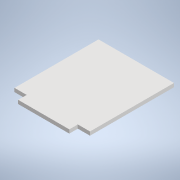
# Autodesk Inventor part: divider 2
Saved by Autodesk Inventor 2022 (Build 260153000, 153)
## iProperties
Created: 2022-05-12
Part Number: divider 2
Material: Generic
Document SubType Name: Modeling
Designer: Jeanette Guo
Density: 1 g/cm^3
Appearance: Default
Author: Jeanette Guo
Autodesk Inventor part; units mm, degrees
ref_plane "YZ Plane" through (0, 0, 0) normal (1, 0, 0) x (0, 1, 0)
ref_plane "XZ Plane" through (0, 0, 0) normal (0, 1, 0) x (-1, 0, 0)
ref_plane "XY Plane" through (0, 0, 0) normal (0, 0, 1) x (1, 0, 0)
sketch "Sketch1" plane through (0, 0, 0) normal (0, 0, 1) x (1, 0, 0)
  line L0 (50, -20) -> (8, -20) projected
  line L1 (8, -17) -> (50, -17) projected
  line L2 (50, -17) -> (50, -20) projected
  line L3 (8, -20) -> (8, -17) projected
  line L4 (50, -17) -> (8, -17)
  line L5 (8, -17) -> (8, -20)
  line L6 (8, -20) -> (50, -20)
  line L7 (50, -20) -> (50, -17)
  point P0 (0, 0)
  constraints: 8 end point, 2 parallel, 1 horizontal, 1 perpendicular
extrude "Extrusion1" add sketch "Sketch1" along normal blind 76
sketch "Sketch2" plane through (50, -20, 0) normal (1, 0, 0) x (0, 0, -1)
  line L0 (-73, 6.5) -> (-73, 16.5) projected
  line L1 (0, 3) -> (-76, 3) projected
  line L2 (0, 0) -> (0, 3) projected
  line L3 (0, 0) -> (-76, 0) projected
  line L4 (-73, 0) -> (0, 0)
  line L5 (0, 0) -> (0, 3)
  line L6 (0, 3) -> (-73, 3)
  line L7 (-73, 3) -> (-73, 0)
  point P0 (0, 20)
  point P1 (-69, 3)
  point P2 (-69, 1.5)
  point P3 (-73, 3)
  constraints: 8 end point, 2 parallel, 2 point on line, 1 horizontal, 1 perpendicular
extrude "Extrusion2" add sketch "Sketch2" along normal blind 10
sketch "Sketch3" plane through (8, -20, 0) normal (-1, 0, 0) x (0, 0, 1)
  line L0 (73, 6.5) -> (73, 16.5) projected
  line L1 (0, 3) -> (0, 0) projected
  line L2 (0, 3) -> (76, 3) projected
  line L3 (73, 3) -> (0, 3)
  line L4 (0, 3) -> (0, 0)
  line L5 (0, 0) -> (73, 0)
  line L6 (73, 0) -> (73, 3)
  point P0 (0, 20)
  point P1 (69, 0)
  point P2 (69, 1.5)
  constraints: 8 end point, 2 parallel, 2 point on line, 1 horizontal, 1 perpendicular
extrude "Extrusion3" add sketch "Sketch3" along normal blind 10
body "Solid1"
